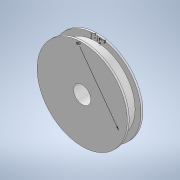
# Autodesk Inventor part: Return_Spool
Saved by Autodesk Inventor 2022 (Build 260153070, 153G)
## iProperties
Created: 2022-03-05
Part Number: Return_Spool
Material: Generic
Document SubType Name: Modeling
Designer: a laptop
Density: 1 g/cm^3
Appearance: Default
Author: a laptop
Autodesk Inventor part; units mm, degrees
ref_plane "YZ Plane" through (0, 0, 0) normal (1, 0, 0) x (0, 1, 0)
ref_plane "XZ Plane" through (0, 0, 0) normal (0, 1, 0) x (-1, 0, 0)
ref_plane "XY Plane" through (0, 0, 0) normal (0, 0, 1) x (1, 0, 0)
sketch "Sketch1" plane through (0, 0, 0) normal (0, 0, 1) x (1, 0, 0)
  circle A0 centre (0, 0) radius 50
  circle A1 centre (0, 0) radius 11
  circle A2 centre (0, 0) radius 57.5
  dimension "d0" = 100
  dimension "d1" = 22
  dimension "d2" = 115
  constraints: 3 centre point, 3 coincident
  measures "d0" diameter of A0
  measures "d1" diameter of A1
  measures "d2" diameter of A2
extrude "Extrusion7" add sketch "Sketch1" along normal blind 17.5 and the other way blind 2.5 contours A0
extrude "Extrusion8" add sketch "Sketch1" along normal blind 17.5 and the other way blind 2.5
extrude "Extrusion9" cut sketch "Sketch1" along normal blind 15 contours A2
extrude "Extrusion10" cut sketch "Sketch1" along normal blind 20 and the other way blind 10 contours A1
sketch "Sketch5" plane through (0, 0, -2.5) normal (0, 0, -1) x (-1, 0, 0)
  circle A0 centre (0, 0) radius 40
  line L0 (0, 40) -> (1, 40)
  line L1 (1, 40) -> (1, 43)
  line L2 (0, 44) -> (0, 40)
  line L3 (7, 46) -> (7, 45)
  line L4 (7, 45) -> (3, 45)
  arc A1 (3, 45) -> (1, 43) centre (3, 43) ccw
  arc A2 (2, 46) -> (0, 44) centre (2, 44) ccw
  line L5 (2, 46) -> (7, 46)
  dimension "d35" = 80
  dimension "d37" = 1
  dimension "d38" = 4
  dimension "d39" = 2
  dimension "d40" = 2
  dimension "d41" = 1
  dimension "d42" = 7
  constraints: 13 end point, 4 point on circle, 4 tangent, 3 perpendicular, 2 centre point, 2 horizontal, 2 vertical alignment, 1 coincident, 1 parallel, 2 other
  measures "d37" distance of L3.start L3.end
  measures "d38" distance of L2.start L0.start
  measures "d39" radius of A1
  measures "d40" radius of A2
  measures "d41" distance between parallel lines of L1 L2
  measures "d42" horizontal distance of L2.start L3.start
extrude "Extrusion11" cut sketch "Sketch5" against normal blind 8
sketch "Sketch6" plane through (0, 0, 0) normal (0, 1, 0) x (-1, 0, 0)
  circle A0 centre (0, 0) radius 4
  dimension "d45" = 8
  constraints: 1 centre point, 1 coincident
  measures "d45" diameter of A0
extrude "Extrusion12" cut sketch "Sketch6" against normal blind 77.25
body "Solid2"
